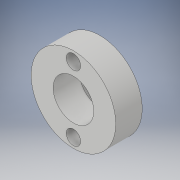
# Autodesk Inventor part: shaft adapter
Saved by Autodesk Inventor 2019 (Build 230136000, 136)
## iProperties
Company: Innovation First, Inc.
Created: 2007-08-24
Part Number: shaft adapter
Material: Generic
Description: STEP AP203
Document SubType Name: Modeling
Designer: User
Density: 1 g/cm^3
Appearance: Default
Sending System: SolidWorks 2006052
Preprocessor: SwSTEP 2.0
Title: SHAFT-3000.STEP
Author: Innovation First, Inc.
Revision Number: ANY
Autodesk Inventor part; units mm, degrees
ref_plane "YZ Plane" through (0, 0, 0) normal (1, 0, 0) x (0, 1, 0)
ref_plane "XZ Plane" through (0, 0, 0) normal (0, 1, 0) x (-1, 0, 0)
ref_plane "XY Plane" through (0, 0, 0) normal (0, 0, 1) x (1, 0, 0)
ref_plane "Work Plane2" through (-0.3779, -1.5875, 39.37) normal (0, 0, 1) x (1, 0, 0)
sketch "Sketch3" plane through (-0.3779, -1.5875, 39.37) normal (0, 0, 1) x (1, 0, 0)
  circle A0 centre (0.3779, 1.5875) radius 10.16
  circle A1 centre (0.3779, 9.4425) radius 1.7272
  circle A2 centre (0.3779, -6.2675) radius 1.7272
  circle A3 centre (0.3779, 1.5875) radius 4.8768
  dimension "d9" = 20.32
  dimension "d10" = 3.4544
  dimension "d11" = 3.4544
  dimension "d12" = 15.7099
  dimension "d13" = 7.8549
  dimension "d14" = 9.7536
  dimension "d16" = 0
  dimension "d26" = 7.8549
  constraints: 4 centre point, 2 coincident
  measures "d9" diameter of A0
  measures "d10" diameter of A1
  measures "d11" diameter of A2
  measures "d12" distance of A2.centre A1.centre
  measures "d13" distance of A0.centre A2.centre
  measures "d14" diameter of A3
  measures "d16" horizontal distance of point (0.378, 1.588) A2.centre
  measures "d26" distance of point (0.378, 1.588) A1.centre
extrude "Extrusion2" add sketch "Sketch3" along normal blind 6.35
sketch "Sketch4" plane through (0, 0, 39.37) normal (0, 0, -1) x (-1, 0, 0)
  circle A0 centre (0, 0) radius 5.715
  dimension "d27" = 11.43
  constraints: 1 centre point, 1 coincident
  measures "d27" diameter of A0
extrude "Extrusion4" add sketch "Sketch4" along normal blind 1.6002
sketch "Sketch5" plane through (0, 0, 37.7698) normal (0, 0, -1) x (-1, 0, 0)
  line L0 (1.5875, -1.5875) -> (-1.5875, -1.5875)
  line L1 (-1.5875, -1.5875) -> (-1.5875, 1.5875)
  line L2 (-1.5875, 1.5875) -> (1.5875, 1.5875)
  line L3 (1.5875, 1.5875) -> (1.5875, -1.5875)
  point P0 (0, 0)
  dimension "d30" = 1.5875
  dimension "d31" = 1.5875
  dimension "d32" = 3.175
  dimension "d33" = 3.175
  constraints: 8 end point, 2 parallel, 1 horizontal, 1 perpendicular
  measures "d30" horizontal distance of point (0, 0) L0.start
  measures "d31" horizontal distance of point (0, 0) L0.start
  measures "d32" distance of L1.end L2.end
  measures "d33" distance between parallel lines of L0 L2
extrude "Extrusion5" cut sketch "Sketch5" against normal through all
equation "\"d13\" = 0.5 * d12"
equation "\"d26\" = d13"
equation "\"d31\" = d30"
equation "\"d33\" = d32"
body "Solid1"
